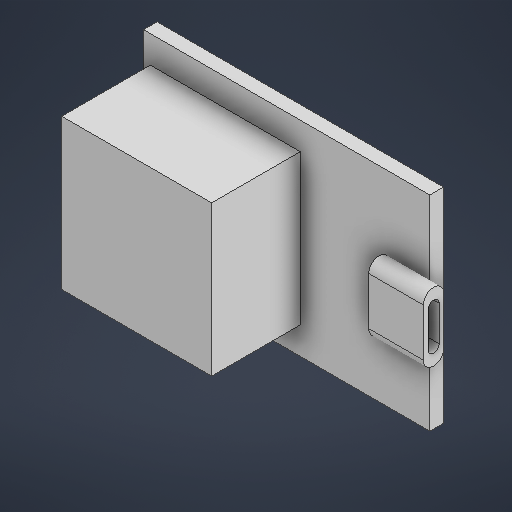
# Autodesk Inventor part: 陀螺仪
Saved by Autodesk Inventor 2025 (Build 290162000, 162)
## iProperties
Created: 2025-01-05
Part Number: 陀螺仪
Material: 常规
Document SubType Name: Modeling
Designer: HZD
Density: 1 g/cm^3
Appearance: 默认
Author: HZD
Autodesk Inventor part; units mm, degrees
ref_plane "YZ Plane" through (0, 0, 0) normal (1, 0, 0) x (0, 1, 0)
ref_plane "XZ Plane" through (0, 0, 0) normal (0, 1, 0) x (-1, 0, 0)
ref_plane "XY Plane" through (0, 0, 0) normal (0, 0, 1) x (1, 0, 0)
sketch "草图1" plane through (0, 0, 0) normal (0, 0, 1) x (1, 0, 0)
  line L0 (21, -15) -> (-21, -15)
  line L1 (-21, -15) -> (-21, 15)
  line L2 (-21, 15) -> (21, 15)
  line L3 (21, 15) -> (21, -15)
  line L4 (21, -15) -> (-21, 15) construction
  line L5 (-21, -15) -> (21, 15) construction
  point P0 (0, 0)
  dimension "d0" = 42
  dimension "d1" = 30
  constraints: 12 end point, 2 midpoint, 2 parallel, 1 horizontal, 1 perpendicular
  measures "d0" distance of L1.end L2.end
  measures "d1" distance of L2.end L0.start
extrude "拉伸1" add sketch "草图1" along normal blind 2
sketch "草图2" plane through (0, 0, 2) normal (0, 0, 1) x (1, 0, 0)
  line L0 (2, -11) -> (-20, -11)
  line L1 (-20, -11) -> (-20, 11)
  line L2 (-20, 11) -> (2, 11)
  line L3 (2, 11) -> (2, -11)
  line L4 (2, -11) -> (-20, 11) construction
  line L5 (-20, -11) -> (2, 11) construction
  line L6 (-21, 15) -> (-21, -15) projected
  point P0 (0, 0)
  point P1 (-9, 0)
  dimension "d4" = 22
  dimension "d5" = 22
  dimension "d6" = 1
  constraints: 12 end point, 2 midpoint, 2 parallel, 1 horizontal, 1 perpendicular
  measures "d4" distance of L2.end L0.start
  measures "d5" distance of L1.end L2.end
  measures "d6" distance between parallel lines of L6 L1
extrude "拉伸2" add sketch "草图2" along normal blind 13
sketch "草图3" plane through (0, 0, 2) normal (0, 0, 1) x (1, 0, 0)
  point P0 (0, 0)
sketch "草图4" plane through (21, -15, 0) normal (1, 0, 0) x (0, 0, -1)
  line L0 (0, 15) -> (-5.9619, 15)
  line L1 (-3.4523, 11.5) -> (-3.4523, 18.5) construction
  line L2 (-1.9523, 11.5) -> (-1.9523, 18.5)
  line L3 (-4.9523, 18.5) -> (-4.9523, 11.5)
  arc A0 (-4.9523, 11.5) -> (-1.9523, 11.5) centre (-3.4523, 11.5) ccw
  arc A1 (-1.9523, 18.5) -> (-4.9523, 18.5) centre (-3.4523, 18.5) ccw
  line L4 (-3.4523, 12.4289) -> (-3.4523, 17.5711) construction
  line L5 (-2.6459, 12.4289) -> (-2.6459, 17.5711)
  line L6 (-4.2587, 17.5711) -> (-4.2587, 12.4289)
  arc A2 (-4.2587, 12.4289) -> (-2.6459, 12.4289) centre (-3.4523, 12.4289) ccw
  arc A3 (-2.6459, 17.5711) -> (-4.2587, 17.5711) centre (-3.4523, 17.5711) ccw
  point P0 (-3.4523, 15)
  point P1 (-3.4523, 10)
  point P2 (-3.4523, 20)
  dimension "d9" = 3
  dimension "d10" = 10
  constraints: 18 end point, 10 point on circle, 8 tangent, 4 centre point, 2 midpoint, 2 parallel, 2 point on line, 1 horizontal, 1 perpendicular
  measures "d9" distance between parallel lines of L2 L3
  measures "d10" distance of point (-3.452, 10) point (-3.452, 20)
extrude "拉伸3" add sketch "草图4" against normal blind 6 contours L2 A0 L3 L0 L6 A2 L5 | L0 L5 A3 L6 L3 A1 L2
extrude "拉伸4" add sketch "草图4" along normal blind 2 contours L2 A0 L3 L0 L6 A2 L5 | L0 L5 A3 L6 L3 A1 L2
sketch "草图5" plane through (15, -15, 0) normal (-1, 0, 0) x (0, 0, 1)
  line L0 (2.6459, 12.4289) -> (2.6459, 17.5711) projected
  arc A0 (4.2587, 17.5711) -> (2.6459, 17.5711) centre (3.4523, 17.5711) ccw projected
  line L1 (4.2587, 17.5711) -> (4.2587, 12.4289) projected
  arc A1 (2.6459, 12.4289) -> (4.2587, 12.4289) centre (3.4523, 12.4289) ccw projected
  line L2 (2, 11.1247) -> (2, 18.8753) projected
  arc A2 (2, 11.1247) -> (4.9523, 11.5) centre (3.4523, 11.5) ccw projected
  line L3 (4.9523, 11.5) -> (4.9523, 18.5) projected
  arc A3 (4.9523, 18.5) -> (2, 18.8753) centre (3.4523, 18.5) ccw projected
  point P0 (0, 15)
extrude "拉伸5" add sketch "草图5" against normal blind 4.25 contours L0 A0 L1 A1 | L2 A3 L3 A2
